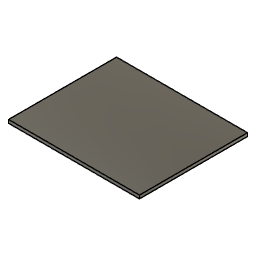
bdn9-exact-plate (Autodesk Fusion 360 design; units mm, degrees)
Autodesk Fusion 360 part; units mm, degrees
sketch "Sketch1" plane through (0, 0, 0) normal (0, 0, 1) x (1, 0, 0)
  line L0 (-1.8548, 0) -> (78.1452, 0)
  line L1 (78.1452, 0) -> (78.1452, 66)
  line L2 (78.1452, 66) -> (-1.8548, 66)
  line L3 (-1.8548, 66) -> (-1.8548, 0)
  dimension "d1" = 80
  dimension "d2" = 66
  constraint horizontal L0
  constraint vertical L1
  constraint horizontal L2
  constraint vertical L3
  measures "d1" distance of L0.start L0.end
  measures "d2" distance of L0.start L2.end
extrude "Extrude1" add sketch "Sketch1" along normal blind 2
